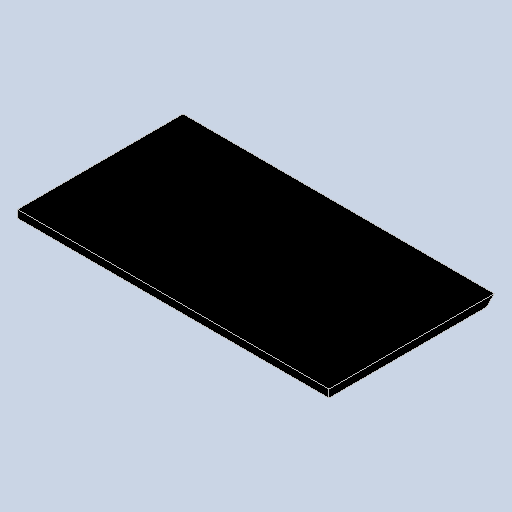
# Autodesk Inventor part: 黒棒
Saved by Autodesk Inventor 2022 (Build 260153000, 153)
## iProperties
Created: 2022-11-24
Part Number: 黒棒
Material: ABS プラスチック
Document SubType Name: Modeling
Designer: tdn82
Density: 1.06 g/cm^3
Appearance: 既定(1)
Author: tdn82
Autodesk Inventor part; units mm, degrees
ref_plane "YZ Plane" through (0, 0, 0) normal (1, 0, 0) x (0, 1, 0)
ref_plane "XZ Plane" through (0, 0, 0) normal (0, 1, 0) x (-1, 0, 0)
ref_plane "XY Plane" through (0, 0, 0) normal (0, 0, 1) x (1, 0, 0)
sketch "スケッチ1" plane through (0, 0, 0) normal (0, 1, 0) x (-1, 0, 0)
  line L0 (0, 0) -> (-80, 0)
  line L1 (-80, 0) -> (-80, -42.5)
  line L2 (-80, -42.5) -> (0, -42.5)
  line L3 (0, -42.5) -> (0, 0)
  dimension "d0" = 80
  dimension "d1" = 42.5
  constraints: 8 end point, 2 parallel, 1 horizontal, 1 perpendicular
  measures "d0" distance of L1.end L2.end
  measures "d1" distance of L2.end L0.start
extrude "押し出し1" add sketch "スケッチ1" along normal blind 2
chamfer "面取り4" distance 2 angle 45 1 edges at (40, 0, -42.5)
